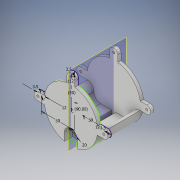
# Autodesk Inventor part: Astra_slot
Saved by Autodesk Inventor 2019 (Build 230136000, 136)
## iProperties
Created: 2019-08-02
Part Number: Astra_slot
Material: Generic
Document SubType Name: Modeling
Designer: leode
Density: 1 g/cm^3
Appearance: Default
Author: leode
Autodesk Inventor part; units mm, degrees
note: some values were not read from the file. Chosen so that the rebuilt part matches the saved one: sketch regions of "Extrusion2".
ref_plane "YZ Plane" through (0, 0, 0) normal (1, 0, 0) x (0, 1, 0)
ref_plane "XZ Plane" through (0, 0, 0) normal (0, 1, 0) x (-1, 0, 0)
ref_plane "XY Plane" through (0, 0, 0) normal (0, 0, 1) x (1, 0, 0)
sketch "Sketch1" plane through (0, 0, 0) normal (0, 0, 1) x (1, 0, 0)
  circle A0 centre (0, 0) radius 40.5
  line L0 (0, 0) -> (0, 50) construction
  arc A1 (6, 50) -> (-6, 50) centre (0, 50) ccw
  line L1 (0, 0) -> (50, 0) construction
  arc A2 (50, -6) -> (50, 6) centre (50, 0) ccw
  line L2 (0, 0) -> (-50, 0) construction
  arc A3 (-50, 6) -> (-50, -6) centre (-50, 0) ccw
  line L3 (-6, 50) -> (-6, 40.0531)
  line L4 (6, 40.0531) -> (6, 50)
  line L5 (-40.0531, 6) -> (-50, 6)
  line L6 (-50, -6) -> (-40.0531, -6)
  line L7 (50, 6) -> (40.0531, 6)
  line L8 (40.0531, -6) -> (50, -6)
  circle A4 centre (-50, 0) radius 1.75
  circle A5 centre (0, 50) radius 1.75
  circle A6 centre (50, 0) radius 1.75
  point P0 (0, 25)
  point P1 (25, 0)
  point P2 (-25, 0)
  dimension "d0" = 81
  dimension "d3" = 50
  dimension "d4" = 12
  dimension "d5" = 50
  dimension "d6" = 12
  dimension "d7" = 50
  dimension "d8" = 12
  dimension "d9" = 3.5
  dimension "d10" = 3.5
  dimension "d11" = 3.5
  constraints: 24 end point, 12 point on circle, 7 centre point, 6 tangent, 4 coincident, 3 midpoint, 3 parallel, 1 perpendicular, 1 point on line, 1 vertical
  measures "d0" diameter of A0
  measures "d3" distance of L0.start L0.end
  measures "d4" diameter of A1
  measures "d5" distance of L0.start L1.end
  measures "d6" diameter of A2
  measures "d7" distance of L0.start L2.end
  measures "d8" diameter of A3
  measures "d9" diameter of A4
  measures "d10" diameter of A5
  measures "d11" diameter of A6
extrude "Extrusion2" add sketch "Sketch1" along normal blind 5
sketch "Sketch2" plane through (0, 0, 5) normal (0, 0, 1) x (1, 0, 0)
  arc A0 (-40.0531, -6) -> (40.0531, -6) centre (0, 0) ccw projected
  line L0 (-40.0531, -6) -> (-40.0531, -6)
  line L1 (-40.0531, -6) -> (-40.0531, -6) construction
  line L2 (-30.0531, -16) -> (-30.0531, -17.1489)
  line L3 (40.0531, -6) -> (40.0531, -6)
  line L4 (30.0531, -16) -> (30.0531, -17.1489)
  arc A1 (-30.0531, -17.1489) -> (-20.0531, -27.1489) centre (-20.0531, -17.1489) ccw
  arc A2 (20.0531, -27.1489) -> (30.0531, -17.1489) centre (20.0531, -17.1489) ccw
  arc A3 (40.0531, -6) -> (30.0531, -16) centre (40.0531, -16) ccw
  arc A4 (-30.0531, -16) -> (-40.0531, -6) centre (-40.0531, -16) ccw
  line L5 (-3, -27.1489) -> (-3, -40.3887)
  line L6 (3, -27.1489) -> (3, -40.3887)
  line L7 (20.0531, -27.1489) -> (3, -27.1489)
  line L8 (-3, -27.1489) -> (-20.0531, -27.1489)
  point P0 (-30.0531, -6)
  point P1 (-30.0531, -27.1489)
  point P2 (30.0531, -6)
  point P3 (30.0531, -27.1489)
  dimension "d16" = 10
  dimension "d17" = 0
  dimension "d18" = 90
  dimension "d19" = 10
  dimension "d20" = 10
  constraints: 18 end point, 12 point on circle, 10 tangent, 6 point on line, 4 centre point, 3 equal radius, 3 horizontal, 1 collinear, 1 perpendicular
  measures "d16" distance of L0.start point (-30.053, -6)
  measures "d17" distance between parallel lines of L0 L1
  measures "d18" angle of L0 L2
  measures "d19" distance of L3.start point (30.053, -6)
  measures "d20" radius of A1
extrude "Extrusion3" add sketch "Sketch2" along normal blind 60
sketch "Sketch3" plane through (0, 0, 65) normal (0, 0, 1) x (1, 0, 0)
  arc A0 (3, -40.3621) -> (-3, -40.3621) centre (0, 0) ccw
  arc A1 (6, 50) -> (-6, 50) centre (0, 50) ccw projected
  line L0 (0, 0) -> (0, 50) construction
  line L1 (6, 0) -> (6, 50)
  line L2 (-6, 50) -> (-6, 0)
  arc A2 (-6, 0) -> (6, 0) centre (0, 0) ccw
  arc A3 (6, 50) -> (-6, 50) centre (0, 50) ccw
  line L3 (0, 0) -> (50, 0) construction
  line L4 (0, 0) -> (50, 0) construction
  line L5 (0, -6) -> (50, -6)
  line L6 (50, 6) -> (0, 6)
  arc A4 (0, 6) -> (0, -6) centre (0, 0) ccw
  arc A5 (50, -6) -> (50, 6) centre (50, 0) ccw
  line L7 (0, 0) -> (-50, 0) construction
  line L8 (0, 6) -> (-50, 6)
  line L9 (-50, -6) -> (0, -6)
  arc A6 (0, -6) -> (0, 6) centre (0, 0) ccw
  arc A7 (-50, 6) -> (-50, -6) centre (-50, 0) ccw
  circle A8 centre (50, 0) radius 1.75
  circle A9 centre (-50, 0) radius 1.75
  circle A10 centre (0, 50) radius 1.75
  line L10 (-3, -40.3887) -> (-3, -36.6883)
  line L11 (3, -36.6883) -> (3, -40.3887)
  arc A11 (3, -36.6883) -> (-3, -36.6883) centre (0, -27.1489) ccw
  point P0 (0, 25)
  point P1 (25, 0)
  point P2 (-25, 0)
  dimension "d26" = 50
  dimension "d27" = 90
  dimension "d28" = 12
  dimension "d29" = 50
  dimension "d30" = 12
  dimension "d31" = 50
  dimension "d32" = 12
  dimension "d33" = 3.5
  dimension "d34" = 3.5
  dimension "d35" = 3.5
  dimension "d45" = 20
  constraints: 30 end point, 16 point on circle, 12 tangent, 11 centre point, 4 coincident, 3 midpoint, 3 parallel, 3 point on line, 2 perpendicular, 1 horizontal, 1 vertical
  measures "d26" distance of L0.start L0.end
  measures "d27" angle of L3 L0
  measures "d28" diameter of A3
  measures "d29" distance of L0.start L4.end
  measures "d30" diameter of A5
  measures "d31" distance of L0.start L7.end
  measures "d32" diameter of A7
  measures "d33" diameter of A8
  measures "d34" diameter of A9
  measures "d35" diameter of A10
  measures "d45" diameter of A11
extrude "Extrusion4" add sketch "Sketch3" along normal blind 5
sketch "Sketch4" plane through (3, -27.1489, 5) normal (0, 1, 0) x (1, 0, 0)
  line L0 (7, -60) -> (0, -60) projected
  line L1 (-6, -60) -> (-13, -60) projected
  line L2 (0, -70) -> (5, -70) projected
  line L3 (5, -70) -> (13, -70) construction
  line L4 (-6, -60) -> (-43.0263, -60) projected
  line L5 (-11, -70) -> (-3, -70) construction
  line L6 (7, -60) -> (-13, -60)
  line L7 (-13, -60) -> (-13, -52)
  line L8 (-13, -52) -> (7, -52)
  line L9 (7, -52) -> (7, -60)
  line L10 (7, -60) -> (-13, -60)
  line L11 (-13, -60) -> (-13, -65)
  line L12 (-13, -65) -> (7, -65)
  line L13 (7, -65) -> (7, -60)
  point P0 (-3, 5)
  point P1 (0, -60)
  dimension "d46" = 8
  dimension "d47" = 20
  dimension "d48" = 5
  constraints: 18 end point, 4 parallel, 3 horizontal, 2 perpendicular, 6 other
  measures "d46" distance of L6.end L7.end
  measures "d47" distance of L12.end L11.end
  measures "d48" distance of L11.end L10.end
extrude "Extrusion5" cut sketch "Sketch4" against normal blind 15
ref_plane "Work Plane1" through (0, 0, 65) normal (-1, 0, 0) x (0, 1, 0)
body "Solid2"
